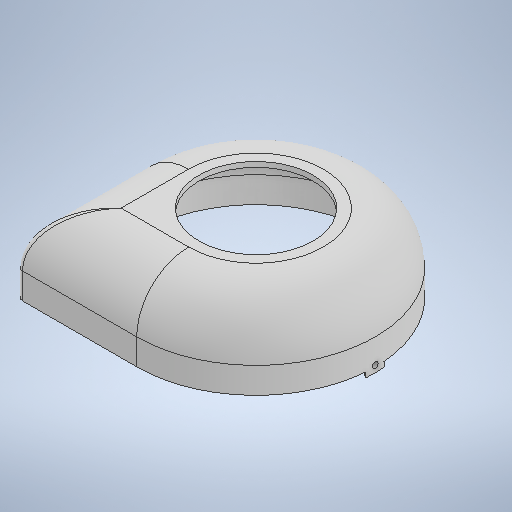
# Autodesk Inventor part: Cylinder Housing_cap_3
Saved by Autodesk Inventor 2025 (Build 290162000, 162)
## iProperties
Created: 2025-10-06
Part Number: Cylinder Housing_cap_3
Material: Generic
Document SubType Name: Modeling
Designer: mumin
Density: 1 g/cm^3
Appearance: Default
Author: mumin
Autodesk Inventor part; units mm, degrees
ref_plane "YZ Plane" through (0, 0, 0) normal (1, 0, 0) x (0, 1, 0)
ref_plane "XZ Plane" through (0, 0, 0) normal (0, 1, 0) x (-1, 0, 0)
ref_plane "XY Plane" through (0, 0, 0) normal (0, 0, 1) x (1, 0, 0)
sketch "Sketch1" plane through (0, 0, 0) normal (0, 1, 0) x (-1, 0, 0)
  arc A0 (0, 115) -> (115, 0) centre (0, 0) ccw
  line L0 (115, 0) -> (115, 110)
  line L1 (110, 115) -> (0, 115)
  arc A1 (115, 110) -> (110, 115) centre (110, 110) ccw
  dimension "d0" = 230
  dimension "d1" = 5
  constraints: 4 end point, 4 point on circle, 2 centre point, 2 tangent, 1 coincident
  measures "d0" diameter of A0
  measures "d1" radius of A1
extrude "Base Shape & Wall" add sketch "Sketch1" along normal blind 75
fillet "Curved Edge" radius 50 4 edges at (81.3173, 75, -81.3173) (-115, 75, 55) (-113.5355, 75, 113.5355) (-55, 75, 115)
shell "Shell" thickness 4.9 removed faces 1 at (-52.6749, 0, -2.0856)
sketch "Sketch2" plane through (0, 75, 0) normal (0, 1, 0) x (1, 0, 0)
  point P0 (0, 0)
  point P1 (0, 0)
  constraints: 1 coincident
hole "Cylinder Hole" at (0, 75, 0) direction (0, -1, 0) diameter 110 end through all
sketch "Sketch3" plane through (0, 0, 0) normal (0, -1, 0) x (1, 0, 0)
  arc A0 (-115, 0) -> (0, 115) centre (0, 0) ccw projected
  line L0 (0, 65) -> (0, 110.1) projected
  line L1 (-110.1, 0) -> (-65, 0) projected
  arc A1 (-110.1, 0) -> (0, 110.1) centre (0, 0) ccw projected
  line L2 (114.6551, 8.9) -> (109.9418, 5.9)
  line L3 (109.9418, -5.9) -> (114.6551, -8.9)
  line L4 (-199.1076, 0) -> (222.9249, 0) projected
  arc A2 (-65, 0) -> (0, 65) centre (0, 0) ccw projected
  point P0 (-55, 0)
  dimension "d13" = 5.9
  dimension "d14" = 8.9
  constraints: 4 end point, 4 point on circle, 2 symmetric about line
  measures "d13" distance from line of L4 L2.end
  measures "d14" distance from line of L4 L2.start
extrude "Front Tab" add sketch "Sketch3" along normal blind 5 contours L3 A1 L4 A0 | L4 A1 L2 A0 picked at (113.1479, -6.9122)
sketch "Sketch4" plane through (0, 0, 0) normal (1, 0, 0) x (0, 1, 0)
  line L0 (0, 0) -> (25, 0) projected
  circle A0 centre (1.5, 0) radius 2.75
  line L1 (-5, 8.9) -> (-5, -8.9) projected
  dimension "d17" = 5.5
  dimension "d18" = 6.5
  constraints: 1 centre point, 1 point on line
  measures "d17" diameter of A0
  measures "d18" distance from line of L1 A0.centre
extrude "Bolt Hole" cut sketch "Sketch4" along normal through all
sketch "Sketch5" plane through (0, 0, 0) normal (0, 0, 1) x (1, 0, 0)
  line L0 (115, 25) -> (-115, 25) projected
  line L1 (110.1, 25) -> (-110.1, 25) projected
  line L2 (-110.1, 0) -> (-110.1, 25) projected
  line L3 (-110.1, 0) -> (-110.1, 25)
  line L4 (-110.1, 25) -> (-112.6, 25)
  line L5 (-110.1, 0) -> (-112.6, 25)
  line L6 (-110.1, 0) -> (-108.0437, 0)
  line L7 (-108.0437, 0) -> (-108.0437, 25)
  point P0 (0, 0)
  point P1 (0, 25)
  dimension "d22" = 2.5
  constraints: 10 end point, 2 point on line, 1 collinear, 1 horizontal, 1 perpendicular
  measures "d22" distance of L4.end L1.end
extrude "Extrusion4" cut sketch "Sketch5" along normal mid plane 15
body "Solid1"
